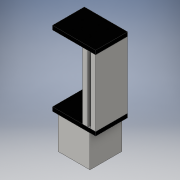
# Autodesk Inventor part: Linear stepper
Saved by Autodesk Inventor 2016 (Build 200138000, 138)
## iProperties
Created: 2015-11-30
Part Number: Linear stepper
Material: Generic
Document SubType Name: Modeling
Designer: Javier
Density: 1 g/cm^3
Appearance: Default
Author: Javier
Autodesk Inventor part; units mm, degrees
sketch "Sketch1" plane through (0, 0, 0) normal (0, 1, 0) x (-1, 0, 0)
  line L0 (24.003, -24.0356) -> (-23.9954, -24.0356)
  line L1 (-23.9954, -24.0356) -> (-23.9954, 23.9628)
  line L2 (-23.9954, 23.9628) -> (24.003, 23.9628)
  line L3 (24.003, 23.9628) -> (24.003, -24.0356)
  point P0 (0, 0)
  dimension "d0" = 47.9984
  constraints: 8 end point, 2 parallel, 2 perpendicular, 1 horizontal
  measures "d0" distance of L0.end L0.start
extrude "Extrusion1" add sketch "Sketch1" along normal blind 48.006
ref_plane "Work Plane1" through (0, 48.006, 0) normal (0, 1, 0) x (-1, 0, 0)
sketch "Sketch2" plane through (0, 48.006, 0) normal (0, 1, 0) x (-1, 0, 0)
  line L0 (32.4891, 23.9092) -> (-32.5095, 23.9092)
  line L1 (-32.5095, 23.9092) -> (-32.5095, -24.0892)
  line L2 (-32.5095, -24.0892) -> (32.4891, -24.0892)
  line L3 (32.4891, -24.0892) -> (32.4891, 23.9092)
  point P0 (0, 0)
  dimension "d6" = 64.9986
  constraints: 8 end point, 2 parallel, 1 horizontal, 1 perpendicular
  measures "d6" distance between parallel lines of L1 L3
extrude "Extrusion2" add sketch "Sketch2" along normal blind 5.9944
sketch "Sketch3" plane through (0, 0, 0) normal (0, 0, 1) x (1, 0, 0)
  line L0 (-32.4891, 54.0004) -> (32.5095, 54.0004) projected
  line L1 (32.5413, 154.0764) -> (12.5515, 154.0764)
  line L2 (12.5515, 154.0764) -> (12.5515, 54.0004)
  line L3 (12.5515, 54.0004) -> (32.5413, 54.0004)
  line L4 (32.5413, 54.0004) -> (32.5413, 154.0764)
  point P0 (0, 0)
  dimension "d12" = 19.9898
  dimension "d13" = 100.076
  constraints: 8 end point, 2 parallel, 1 horizontal, 1 perpendicular, 1 point on line
  measures "d12" distance of L1.start L1.end
  measures "d13" distance between parallel lines of L3 L1
extrude "Extrusion3" add sketch "Sketch3" along normal mid plane 48.006
ref_plane "Work Plane2" through (0, 0, 24.003) normal (0, 0, 1) x (1, 0, 0)
ref_plane "Work Plane3" through (0, 0, -24.003) normal (0, 0, 1) x (1, 0, 0)
sketch "Sketch4" plane through (0, 0, 24.003) normal (0, 0, 1) x (1, 0, 0)
  line L0 (20.6375, 157.1625) -> (25.4, 157.1625)
  line L1 (25.4, 157.1625) -> (25.4, 53.975)
  line L2 (25.4, 53.975) -> (20.6375, 53.975)
  line L3 (20.6375, 53.975) -> (20.6375, 157.1625)
  line L4 (12.5515, 154.0764) -> (12.5515, 54.0004) projected
  point P0 (0, 0)
  dimension "d24" = 4.7625
  dimension "d25" = 8.086
  constraints: 8 end point, 2 parallel, 1 horizontal, 1 perpendicular
  measures "d24" distance between parallel lines of L1 L3
  measures "d25" distance between parallel lines of L3 L4
extrude "Extrusion4" cut sketch "Sketch4" against normal blind 5.08
sketch "Sketch6" plane through (0, 0, -24.003) normal (0, 0, 1) x (1, 0, 0)
  line L0 (20.6375, 53.975) -> (20.6375, 154.0764) projected
  line L1 (25.4, 155.575) -> (20.6375, 155.575)
  line L2 (20.6375, 155.575) -> (20.6375, 53.975)
  line L3 (20.6375, 53.975) -> (25.4, 53.975)
  line L4 (25.4, 53.975) -> (25.4, 155.575)
  point P0 (0, 0)
  constraints: 8 end point, 2 parallel, 1 horizontal, 1 perpendicular
extrude "Extrusion6" cut sketch "Sketch6" along normal blind 5.08
ref_plane "Work Plane4" through (0, 154.178, 0) normal (0, 1, 0) x (-1, 0, 0)
sketch "Sketch7" plane through (0, 154.178, 0) normal (0, 1, 0) x (-1, 0, 0)
  line L0 (-32.5413, 24.003) -> (-32.5413, -24.003) projected
  line L1 (-32.5095, -24.0892) -> (32.4891, -24.0892) projected
  line L2 (-32.5413, 24.003) -> (32.4891, 24.003)
  line L3 (32.4891, 24.003) -> (32.4891, -24.0892)
  line L4 (32.4891, -24.0892) -> (-32.5413, -24.0892)
  line L5 (-32.5413, -24.0892) -> (-32.5413, 24.003)
  point P0 (0, 0)
  constraints: 8 end point, 2 parallel, 1 horizontal, 1 perpendicular
extrude "Extrusion7" add sketch "Sketch7" along normal blind 5.9944
body "Solid1"
